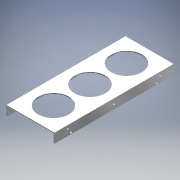
# Autodesk Inventor part: Mottor Protection Piece
Saved by Autodesk Inventor 2019 (Build 230136000, 136)
## iProperties
Created: 2019-11-02
Part Number: Mottor Protection Piece
Material: Aluminum 6061
Document SubType Name: Modeling
Designer: admin
Density: 2.7 g/cm^3
Appearance: Aluminum - Flat
Mass: 284.971 g
Surface Area: 1078.14 cm^2
Volume: 105.545 cm^3
Author: admin
Autodesk Inventor part; units mm, degrees
ref_plane "YZ Plane" through (0, 0, 0) normal (1, 0, 0) x (0, 1, 0)
ref_plane "XZ Plane" through (0, 0, 0) normal (0, 1, 0) x (-1, 0, 0)
ref_plane "XY Plane" through (0, 0, 0) normal (0, 0, 1) x (1, 0, 0)
sketch "Sketch1" plane through (0, 0, 0) normal (0, 0, 1) x (1, 0, 0)
  line L0 (0, 0) -> (0, 25)
  line L1 (0, 25) -> (125, 25)
  line L2 (125, 25) -> (125, 0)
  line L3 (123, 0) -> (123, 23)
  line L4 (123, 23) -> (2, 23)
  line L5 (2, 23) -> (2, 0)
  line L6 (0, 0) -> (2, 0)
  line L7 (123, 0) -> (125, 0)
  dimension "d0" = 25
  dimension "d1" = 125
  dimension "d2" = 25
  dimension "d3" = 2
  constraints: 16 end point, 4 perpendicular, 1 collinear, 1 horizontal, 1 vertical, 2 other
  measures "d0" distance of L0.start L0.end
  measures "d1" distance of L0.end L1.end
  measures "d2" distance of L1.end L2.end
  measures "d3" distance between parallel lines of L1 L4
extrude "Extrusion1" add sketch "Sketch1" along normal mid plane 310
sketch "Sketch2" plane through (125, 0, 155) normal (1, 0, 0) x (0, 0, -1)
  line L0 (-37.1806, -32.4891) -> (-16.9173, -51.5906) projected
  arc A0 (-19.2971, -56.7563) -> (-16.9173, -51.5906) centre (-18.9751, -53.7736) ccw projected
  line L1 (-19.2971, -56.7563) -> (-50.7109, -53.3649) projected
  arc A1 (-50.7109, -53.3649) -> (-55.7198, -43.3108) centre (-69.9997, -56.6998) ccw projected
  line L2 (-55.7198, -43.3108) -> (-48.1647, -31.8699) projected
  arc A2 (-48.1647, -31.8699) -> (-37.1806, -32.4891) centre (-41.913, -18.7038) ccw projected
  line L3 (-75.1262, -21.5392) -> (-58.4909, -21.5392) projected
  arc A3 (-55.6611, -23.5431) -> (-58.4909, -21.5392) centre (-58.4909, -24.5392) ccw projected
  arc A4 (-55.6611, -23.5431) -> (-54.0721, -26.7404) centre (-41.913, -18.7038) ccw projected
  arc A5 (-54.1495, -30.1604) -> (-54.0721, -26.7404) centre (-56.5748, -28.3946) ccw projected
  line L4 (-54.1495, -30.1604) -> (-59.4289, -37.4114) projected
  arc A6 (-62.9366, -38.4435) -> (-59.4289, -37.4114) centre (-61.8542, -35.6456) ccw projected
  arc A7 (-62.9366, -38.4435) -> (-89.5451, -57.7757) centre (-69.9997, -56.6998) ccw projected
  arc A8 (-91.9678, -60.8854) -> (-89.5451, -57.7757) centre (-92.5406, -57.9406) ccw projected
  arc A9 (-94.9634, -58.047) -> (-91.9678, -60.8854) centre (-91.9678, -57.8854) ccw projected
  arc A10 (-90.8616, -42.9236) -> (-94.9634, -58.047) centre (-69.9997, -56.6998) ccw projected
  line L5 (-90.8616, -42.9236) -> (-77.6297, -22.886) projected
  arc A11 (-75.1262, -21.5392) -> (-77.6297, -22.886) centre (-75.1262, -24.5392) ccw projected
  line L6 (14.2318, -42.1167) -> (14.5019, -34.4151) projected
  arc A12 (16.192, -31.8204) -> (14.5019, -34.4151) centre (17.5, -34.5202) ccw projected
  arc A13 (16.192, -31.8204) -> (22.7889, -25.3881) centre (9.837, -18.7038) ccw projected
  arc A14 (25.4548, -23.764) -> (22.7889, -25.3881) centre (25.4548, -26.764) ccw projected
  line L7 (25.4548, -23.764) -> (32.9732, -23.764) projected
  arc A15 (35.8062, -27.7509) -> (32.9732, -23.764) centre (32.9732, -26.764) ccw projected
  arc A16 (20.9479, -43.8593) -> (35.8062, -27.7509) centre (9.837, -18.7038) ccw projected
  line L8 (20.9479, -43.8593) -> (18.4421, -44.9661) projected
  arc A17 (14.2318, -42.1167) -> (18.4421, -44.9661) centre (17.23, -42.2218) ccw projected
  arc A18 (-58.2766, -72.3762) -> (-51.79, -63.8823) centre (-69.9997, -56.6998) ccw projected
  arc A19 (-48.5739, -62.0133) -> (-51.79, -63.8823) centre (-48.9993, -64.983) ccw projected
  line L9 (-48.5739, -62.0133) -> (-37.4758, -63.6029) projected
  arc A20 (-36.689, -69.3169) -> (-37.4758, -63.6029) centre (-37.9011, -66.5726) ccw projected
  line L10 (-36.689, -69.3169) -> (-55.2679, -77.5229) projected
  arc A21 (-58.2766, -72.3762) -> (-55.2679, -77.5229) centre (-56.48, -74.7787) ccw projected
  line L11 (-76.5265, -76.5449) -> (-76.5468, -78.0792) projected
  arc A22 (-79.2898, -79.9096) -> (-76.5468, -78.0792) centre (-78.5466, -78.0528) ccw projected
  arc A23 (-88.4428, -73.5774) -> (-79.2898, -79.9096) centre (-69.9997, -56.6998) ccw projected
  arc A24 (-86.9673, -70.2272) -> (-88.4428, -73.5774) centre (-86.9673, -72.2272) ccw projected
  line L12 (-86.9673, -70.2272) -> (-84.9791, -70.2272) projected
  arc A25 (-83.5905, -70.7878) -> (-84.9791, -70.2272) centre (-84.9791, -72.2272) ccw projected
  arc A26 (-83.5905, -70.7878) -> (-77.7359, -74.6812) centre (-69.9997, -56.6998) ccw projected
  arc A27 (-76.5265, -76.5449) -> (-77.7359, -74.6812) centre (-78.5263, -76.5184) ccw projected
  line L13 (14.5694, -2.9211) -> (14.5694, 4.544) projected
  arc A28 (18.5162, 7.3907) -> (14.5694, 4.544) centre (17.5694, 4.544) ccw projected
  arc A29 (35.8062, -9.6566) -> (18.5162, 7.3907) centre (9.837, -18.7038) ccw projected
  arc A30 (32.9732, -13.6436) -> (35.8062, -9.6566) centre (32.9732, -10.6436) ccw projected
  line L14 (32.9732, -13.6436) -> (25.4548, -13.6436) projected
  arc A31 (22.7889, -12.0194) -> (25.4548, -13.6436) centre (25.4548, -10.6436) ccw projected
  arc A32 (22.7889, -12.0194) -> (16.2495, -5.6152) centre (9.837, -18.7038) ccw projected
  arc A33 (14.5694, -2.9211) -> (16.2495, -5.6152) centre (17.5694, -2.9211) ccw projected
  line L15 (-41.913, 8.7962) -> (-41.4236, 8.7962) projected
  arc A34 (-38.6116, 4.7508) -> (-41.4236, 8.7962) centre (-41.4236, 5.7962) ccw projected
  line L16 (-38.6116, 4.7508) -> (-41.2346, -2.3042) projected
  arc A35 (-43.6823, -4.2366) -> (-41.2346, -2.3042) centre (-44.0465, -1.2588) ccw projected
  arc A36 (-43.6823, -4.2366) -> (-55.6611, -13.8645) centre (-41.913, -18.7038) ccw projected
  arc A37 (-58.4909, -15.8684) -> (-55.6611, -13.8645) centre (-58.4909, -12.8684) ccw projected
  line L17 (-58.4909, -15.8684) -> (-67.4194, -15.8684) projected
  arc A38 (-69.9228, -11.2152) -> (-67.4194, -15.8684) centre (-67.4194, -12.8684) ccw projected
  line L18 (-69.9228, -11.2152) -> (-64.861, -3.5499) projected
  arc A39 (-41.913, 8.7962) -> (-64.861, -3.5499) centre (-41.913, -18.7038) ccw projected
  line L19 (-27.8509, -22.5363) -> (-4.225, -22.5363) projected
  arc A40 (-4.225, -22.5363) -> (3.4806, -31.8196) centre (9.837, -18.7038) ccw projected
  arc A41 (5.089, -35.221) -> (3.4806, -31.8196) centre (2.1722, -34.5193) ccw projected
  line L20 (5.089, -35.221) -> (1.9288, -48.3575) projected
  arc A42 (-2.753, -50.0817) -> (1.9288, -48.3575) centre (-0.988, -47.6558) ccw projected
  line L21 (-2.753, -50.0817) -> (-31.6524, -29.0552) projected
  arc A43 (-31.6524, -29.0552) -> (-27.8509, -22.5363) centre (-41.913, -18.7038) ccw projected
  line L22 (-6.3555, -14.8713) -> (-25.7205, -14.8713) projected
  arc A44 (-28.4845, -13.0375) -> (-25.7205, -14.8713) centre (-25.7205, -11.8713) ccw projected
  arc A45 (-28.4845, -13.0375) -> (-34.5474, -6.1268) centre (-41.913, -18.7038) ccw projected
  arc A46 (-35.6733, -2.1167) -> (-34.5474, -6.1268) centre (-33.0314, -3.5381) ccw projected
  line L23 (-35.6733, -2.1167) -> (-30.6515, 7.2176) projected
  arc A47 (-28.0096, 8.7962) -> (-30.6515, 7.2176) centre (-28.0096, 5.7962) ccw projected
  line L24 (-28.0096, 8.7962) -> (-0.3099, 8.7962) projected
  arc A48 (2.6901, 5.7962) -> (-0.3099, 8.7962) centre (-0.3099, 5.7962) ccw projected
  line L25 (2.6901, 5.7962) -> (2.6901, -4.3539) projected
  arc A49 (1.4221, -6.8034) -> (2.6901, -4.3539) centre (-0.3099, -4.3539) ccw projected
  arc A50 (1.4221, -6.8034) -> (-3.5915, -13.0375) centre (9.837, -18.7038) ccw projected
  arc A51 (-6.3555, -14.8713) -> (-3.5915, -13.0375) centre (-6.3555, -11.8713) ccw projected
  circle A52 centre (-81.913, -5.781) radius 2.75 projected
  circle A53 centre (7.837, -58.4172) radius 2.75 projected
  circle A54 centre (-19.913, 17.776) radius 2.75 projected
  circle A55 centre (-109.9997, -47.6996) radius 2.75 projected
  circle A56 centre (43.4223, 4.8129) radius 2.75 projected
  line L26 (-25.906, 18.0659) -> (-40.1014, 18.7524) projected
  arc A57 (-40.1014, 18.7524) -> (-73.2057, 1.9606) centre (-41.913, -18.7038) ccw projected
  line L27 (-73.2057, 1.9606) -> (-74.4501, 0.0761) projected
  arc A58 (-78.6067, -0.7742) -> (-82.3668, 0.2018) centre (-81.913, -5.781) ccw projected
  line L28 (-85.6456, -16.8777) -> (-99.2063, -37.4131) projected
  arc A59 (-104.9997, -56.6996) -> (-54.959, -88.3032) centre (-69.9997, -56.6998) ccw projected
  arc A60 (-113.4192, -52.6298) -> (-109.9997, -53.6996) centre (-109.9997, -47.6996) ccw projected
  line L29 (-109.9997, -53.6996) -> (-107.9997, -53.6996) projected
  arc A61 (-99.2063, -37.4131) -> (-100.1023, -38.8439) centre (-69.9997, -56.6998) ccw projected
  line L30 (-54.959, -88.3032) -> (2.4193, -60.9957) projected
  arc A62 (2.4193, -60.9957) -> (13.2548, -55.8388) centre (7.837, -58.4172) ccw projected
  line L31 (13.2548, -55.8388) -> (24.8778, -50.3072) projected
  arc A63 (24.8778, -50.3072) -> (42.845, -7.0644) centre (9.837, -18.7038) ccw projected
  line L32 (42.845, -7.0644) -> (48.4494, 1.5375) projected
  arc A64 (48.4494, 1.5375) -> (42.0639, 10.6571) centre (43.4223, 4.8129) ccw projected
  line L33 (42.0639, 10.6571) -> (32.0639, 8.3327) projected
  arc A65 (32.0639, 8.3327) -> (11.5279, 16.2554) centre (9.837, -18.7038) ccw projected
  line L34 (11.5279, 16.2554) -> (-13.92, 17.4862) projected
  arc A66 (-13.92, 17.4862) -> (-25.906, 18.0659) centre (-19.913, 17.776) ccw projected
  circle A67 centre (-69.9997, -56.6998) radius 9.575 projected
  circle A68 centre (-41.913, -18.7038) radius 9.575 projected
  circle A69 centre (9.837, -18.7038) radius 9.575 projected
  circle A70 centre (35, 17) radius 2.75
  circle A71 centre (155, 12.5) radius 2.75
  line L35 (155, 0) -> (155, 25)
  line L36 (0, 25) -> (310, 25) projected
  line L37 (0, 0) -> (0, 25) projected
  circle A72 centre (266.5777, 4.8129) radius 2.75
  circle A73 centre (275, 17) radius 2.75
  circle A74 centre (155, 12.5) radius 2.75
  circle A75 centre (-106.7656, -26.4398) radius 1.65 projected
  arc A76 (-104.9997, -56.6996) -> (-107.9997, -53.6996) centre (-107.9997, -56.6996) ccw projected
  arc A77 (-78.6067, -0.7742) -> (-74.4501, 0.0761) centre (-76.9535, 1.7293) ccw projected
  line L38 (-82.3668, 0.2018) -> (-122.8325, -2.8676) projected
  arc A78 (-122.8325, -2.8676) -> (-132.7182, -39.2443) centre (-121.3198, -22.8103) ccw projected
  line L39 (-132.7182, -39.2443) -> (-113.4192, -52.6298) projected
  circle A79 centre (-131.7402, -33.5999) radius 1.65 projected
  circle A80 centre (-121.3198, -22.8103) radius 10.5 projected
  circle A81 centre (-125.4537, -8.3911) radius 1.65 projected
  line L40 (-104.3923, -39.7785) -> (-104.8988, -39.4272) projected
  arc A82 (-105.5539, -35.1162) -> (-104.8988, -39.4272) centre (-103.189, -36.9621) ccw projected
  arc A83 (-105.5539, -35.1162) -> (-102.1972, -16.9514) centre (-121.3198, -22.8103) ccw projected
  arc A84 (-99.5557, -13.0811) -> (-102.1972, -16.9514) centre (-99.3288, -16.0725) ccw projected
  line L41 (-99.5557, -13.0811) -> (-88.3759, -12.2331) projected
  arc A85 (-85.6456, -16.8777) -> (-88.3759, -12.2331) centre (-88.149, -15.2245) ccw projected
  arc A86 (-104.3923, -39.7785) -> (-100.1023, -38.8439) centre (-102.6826, -37.3134) ccw projected
  point P0 (-69.9997, -56.6998)
  point P1 (-69.9997, -56.6998)
  dimension "d6" = 5.5
  dimension "d7" = 5.5
  dimension "d8" = 8
  dimension "d9" = 12.5
  dimension "d10" = 35
  constraints: 5 centre point, 2 end point, 2 midpoint, 2 symmetric about line, 3 other
  measures "d6" diameter of A70
  measures "d7" diameter of A71
  measures "d8" distance from line of L36 A70.centre
  measures "d9" distance from line of L36 A71.centre
  measures "d10" distance from line of L37 A70.centre
extrude "Extrusion2" cut sketch "Sketch2" against normal blind 205.75 contours A56 | A70 | A71 L35 | L35 A71 | A72 | A73
sketch "Sketch3" plane through (0, 25, 155) normal (0, 1, 0) x (1, 0, 0)
  circle A0 centre (62.5, 60) radius 40
  line L0 (125, 0) -> (125, 310) projected
  line L1 (125, 0) -> (0, 0) projected
  circle A1 centre (62.5, 250) radius 40
  line L2 (0, 310) -> (125, 310) projected
  circle A2 centre (62.5, 155) radius 40
  point P0 (0, 155)
  dimension "d13" = 80
  dimension "d14" = 62.5
  dimension "d15" = 60
  dimension "d16" = 80
  dimension "d17" = 62.5
  dimension "d18" = 60
  dimension "d19" = 80
  dimension "d20" = 62.5
  dimension "d21" = 155
  constraints: 3 centre point
  measures "d13" diameter of A0
  measures "d14" distance from line of L0 A0.centre
  measures "d15" distance from line of L1 A0.centre
  measures "d16" diameter of A1
  measures "d17" distance from line of L0 A1.centre
  measures "d18" distance from line of L2 A1.centre
  measures "d19" diameter of A2
  measures "d20" distance from line of L0 A2.centre
  measures "d21" distance from line of L2 A2.centre
extrude "Extrusion3" cut sketch "Sketch3" against normal blind 10
body "Solid1"
